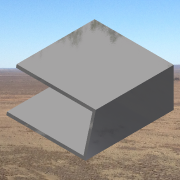
# Autodesk Inventor part: 2p1rim1
Saved by Autodesk Inventor 2013 SP2 (Build 170200200, 200)
## iProperties
Company: HERA Project
Created: 2013-12-03
Part Number: 2p1rim1
Material: Steel, Galvanized
Document SubType Name: Modeling
Designer: David DeBoer
Mass: 492.101 g
Surface Area: 430.611 cm^2
Volume: 62.688 cm^3
Density: 7.85 g/cm^3
Description: end horizontal rim holder 1
Author: David DeBoer
Autodesk Inventor part; units mm, degrees
ref_plane "YZ Plane" through (0, 0, 0) normal (1, 0, 0) x (0, 1, 0)
ref_plane "XZ Plane" through (0, 0, 0) normal (0, 1, 0) x (-1, 0, 0)
ref_plane "XY Plane" through (0, 0, 0) normal (0, 0, 1) x (1, 0, 0)
sketch "Sketch1" plane through (0, 0, 0) normal (0, 0, 1) x (1, 0, 0)
  line L0 (0, 0) -> (88.9, 0)
  line L1 (88.9, 0) -> (88.9, 38.1)
  line L2 (88.9, 38.1) -> (0, 38.1)
  line L3 (0, 38.1) -> (0, 0)
  line L4 (-3.048, 41.148) -> (91.948, 41.148)
  line L5 (91.948, 41.148) -> (91.948, -3.048)
  line L6 (91.948, -3.048) -> (-3.048, -3.048)
  line L7 (-3.048, -3.048) -> (-3.048, 41.148)
  dimension "d0" = 88.9
  dimension "d1" = 38.1
  dimension "d2" = 3.048
  constraints: 16 end point, 4 parallel, 2 perpendicular, 1 horizontal, 3 other
  measures "d0" distance of L0.start L0.end
  measures "d1" distance of L2.end L0.start
  measures "d2" distance between parallel lines of L4 L2
extrude "Extrusion1" add sketch "Sketch1" along normal blind 101.6
ref_plane "Work Plane2" through (-3.048, 41.148, 101.6) normal (0, 0.258819, 0.9659258) x (-1, 0, 0)
sketch "Sketch3" plane through (-3.048, 41.148, 101.6) normal (0, 0.258819, 0.9659258) x (-1, 0, 0)
  line L0 (-130.175, -76.2) -> (53.975, -76.2)
  line L1 (53.975, -76.2) -> (53.975, 57.15)
  line L2 (53.975, 57.15) -> (-130.175, 57.15)
  line L3 (-130.175, 57.15) -> (-130.175, -76.2)
  point P0 (-3.048, 13.4499)
  constraints: 8 end point, 2 parallel, 1 horizontal, 1 perpendicular
extrude "Extrusion3" cut sketch "Sketch3" against normal blind 12.7
sketch "Sketch5" plane through (-3.048, -3.048, 0) normal (-1, 0, 0) x (0, 0, 1)
  line L0 (100.2943, 0) -> (88.452, 44.196) projected
  line L1 (0, 44.196) -> (88.452, 44.196) projected
  line L2 (0, 0) -> (0, 44.196) projected
  line L3 (0, 0) -> (100.2943, 0) projected
  point P0 (0, 3.048)
extrude "Extrusion5" cut sketch "Sketch5" against normal blind 5.08
body "Solid1"
